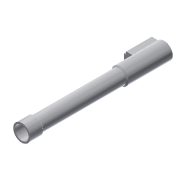
# Autodesk Inventor part: PP-12
Saved by Autodesk Inventor 2022 (Build 260148000, 148)
## iProperties
Created: 2008-09-23
Part Number: PP-12
Document SubType Name: Modeling
Designer: Mark Flayler
Mass: 0.841605 g
Surface Area: 31.0888 cm^2
Volume: 0.793967 cm^3
Density: 1.06 g/cm^3
Material: ABS Plastic
Description: UPPER SHAFT
Appearance: Smooth - White
Author: Mark Flayler
Autodesk Inventor part; units mm, degrees
ref_plane "XZ Plane" through (0, 0, 0) normal (0, 1, 0) x (-1, 0, 0)
ref_plane "XY Plane" through (0, 0, 0) normal (0, 0, 1) x (1, 0, 0)
sketch "Sketch1" plane through (0, 0, 0) normal (0, 0, 1) x (1, 0, 0)
  line L0 (0, 0) -> (0, 66.5)
  line L1 (3.2, 0) -> (4, 0)
  line L2 (4, 0) -> (4, 5.9)
  line L3 (4, 5.9) -> (3.4, 6.5)
  line L4 (3.4, 6.5) -> (3.4, 45.3)
  line L5 (3.4, 45.3) -> (4, 45.9)
  line L6 (4, 45.9) -> (4, 66.5)
  line L7 (4, 66.5) -> (3.2, 66.5)
  line L8 (3.2, 66.5) -> (3.2, 0)
  dimension "d0" = 45
  dimension "d1" = 45
  dimension "d2" = 6.4
  dimension "d3" = 8
  dimension "d4" = 6.5
  dimension "d5" = 45.3
  dimension "d6" = 66.5
  dimension "d7" = 6.8
  constraints: 18 end point, 3 perpendicular, 2 collinear, 2 horizontal alignment, 2 parallel, 1 coincident, 1 vertical
  measures "d0" angle of L4 L3
  measures "d1" angle of L4 L5
  measures "d2" diameter of L8 L0
  measures "d3" diameter of L2 L0
  measures "d4" vertical distance of point (0, 0) L3.end
  measures "d5" vertical distance of point (0, 0) L4.end
  measures "d6" distance from line of point (0, 0) L7
  measures "d7" diameter of L4 L0
revolve "Revolution1" add sketch "Sketch1" angle 360 about axis through (0, 0, 0) along (0, 1, 0)
ref_plane "Work Plane1" through (-6.76, 0, 0) normal (-1, 0, 0) x (0, -1, 0)
sketch "Sketch2" plane through (-6.76, 0, 0) normal (-1, 0, 0) x (0, -1, 0)
  line L0 (-65.7, 1.5) -> (-54.5, 1.5)
  line L1 (-54.5, 1.5) -> (-54.5, -1.5)
  line L2 (-54.5, -1.5) -> (-65.7, -1.5)
  line L3 (-65.7, -1.5) -> (-65.7, 1.5)
  line L4 (-65.7, 2.75) -> (-54.5, 2.75)
  line L5 (-54.5, 2.75) -> (-54.5, -2.75)
  line L6 (-54.5, -2.75) -> (-65.7, -2.75)
  line L7 (-65.7, -2.75) -> (-65.7, 2.75)
  line L8 (13.7787, 0) -> (-82.6723, 0) projected
  line L9 (0, -4) -> (0, 4) projected
  dimension "d10" = 54.5
  dimension "d11" = 65.7
  dimension "d12" = 5.5
  dimension "d13" = 3
  constraints: 16 end point, 4 parallel, 2 collinear, 2 horizontal, 2 perpendicular, 2 other
  measures "d10" distance between parallel lines of L5 L9
  measures "d11" distance between parallel lines of L7 L9
  measures "d12" distance between parallel lines of L4 L6
  measures "d13" distance between parallel lines of L0 L2
extrude "Extrusion1" add sketch "Sketch2" against normal up to surface
extrude "Extrusion2" cut sketch "Sketch2" against normal blind 1 contours L7 L4 L5 L0 | L2 L5 L6 L7
sketch "Sketch3" plane through (-5.76, 0, 0) normal (-1, 0, 0) x (0, 0, 1)
  line L0 (-1.5, 65.7) -> (-1.5, 54.5) projected
  line L1 (-2.75, 65.7) -> (-1.5, 65.7) projected
  line L2 (-2.75, 54.5) -> (-2.75, 65.7) projected
  line L3 (-1.5, 54.5) -> (-2.75, 54.5) projected
  line L4 (1.5, 54.5) -> (1.5, 65.7) projected
  line L5 (2.75, 54.5) -> (1.5, 54.5) projected
  line L6 (2.75, 65.7) -> (2.75, 54.5) projected
  line L7 (1.5, 65.7) -> (2.75, 65.7) projected
  line L8 (-4, 66.5) -> (4, 66.5) projected
  line L9 (2.75, 65.7) -> (-2.75, 65.7)
  line L10 (-2.75, 65.7) -> (-2.75, 66.5)
  line L11 (-2.75, 66.5) -> (2.75, 66.5)
  line L12 (2.75, 66.5) -> (2.75, 65.7)
  constraints: 8 end point, 2 parallel, 1 horizontal, 1 perpendicular, 1 point on line
extrude "Extrusion3" add sketch "Sketch3" against normal up to surface contours L1 L10 L8 L12 L7 L9
sketch "Sketch4" plane through (0, 66.5, 0) normal (0, 1, 0) x (1, 0, 0)
  line L0 (-5.76, 1.5) -> (-5.76, 2.75) projected
  line L1 (-5.76, 2.25) -> (-4.06, 2.25)
  line L2 (-4.06, 2.25) -> (-4.06, -2.25)
  line L3 (-4.06, -2.25) -> (-5.76, -2.25)
  line L4 (-5.76, -2.75) -> (-5.76, 2.75) projected
  line L5 (-4.76, 2.25) -> (-4.76, -2.25)
  line L6 (-8.912, 0) -> (6.152, 0) projected
  line L7 (-5.76, 2.25) -> (-5.76, -2.25)
  point P0 (0, 0)
  dimension "d20" = 4.06
  dimension "d21" = 4.76
  dimension "d22" = 4.5
  constraints: 10 end point, 5 point on line, 2 parallel, 2 perpendicular, 1 collinear, 1 other
  measures "d20" distance from line of L2 point (0, 0)
  measures "d21" distance from line of L5 point (0, 0)
  measures "d22" distance between parallel lines of L3 L1
extrude "Extrusion4" cut sketch "Sketch4" against normal up to surface (0.8 mm away) contours L0 L1 L5 L6 L4 | L6 L5 L3 L4
extrude "Extrusion5" cut sketch "Sketch4" against normal blind 9 contours L1 L2 L6 L5 | L6 L2 L3 L5
equation "\"d1\" = d0"
body "Solid1"
